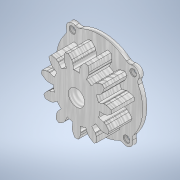
# Autodesk Inventor part: ｍ2歯数10ギアF有d6
Saved by Autodesk Inventor 2020.2 (Build 242310000, 310)
## iProperties
Created: 2020-02-29
Part Number: ｍ2歯数10ギアF有d6
Material: アルミニウム 7075
Document SubType Name: Modeling
Designer: aoyam
Density: 2.81 g/cm^3
Appearance: サテン - ブラシ仕上げ 重厚
Author: aoyam
Autodesk Inventor part; units mm, degrees
ref_plane "YZ Plane" through (0, 0, 0) normal (1, 0, 0) x (0, 1, 0)
ref_plane "XZ Plane" through (0, 0, 0) normal (0, 1, 0) x (-1, 0, 0)
ref_plane "XY Plane" through (0, 0, 0) normal (0, 0, 1) x (1, 0, 0)
sketch "スケッチ1" plane through (0, 0, 0) normal (0, 0, 1) x (1, 0, 0)
  arc A0 (3.44, 13.5335) -> (3.3718, 13.2916) centre (4.6302, 13.067) ccw
  arc A1 (3.8401, 14.2933) -> (3.44, 13.5335) centre (6.7686, 12.2662) ccw
  arc A2 (5.1311, 15.6698) -> (3.8401, 14.2933) centre (9.0569, 10.6941) ccw
  arc A3 (0.735, 13.2916) -> (0.6667, 13.5335) centre (-0.5235, 13.067) ccw
  arc A4 (0.6667, 13.5335) -> (0.2666, 14.2933) centre (-2.6619, 12.2662) ccw
  arc A5 (0.2666, 14.2933) -> (-1.0244, 15.6698) centre (-4.9502, 10.6941) ccw
  arc A6 (3.1375, 11.4699) -> (0.9692, 11.4699) centre (2.0534, 3.0394) ccw
  arc A7 (-1.0244, 15.6698) -> (-2.186, 15.3287) centre (2.0534, 3.0394) ccw
  line L0 (3.1375, 11.4699) -> (3.3718, 13.2916)
  line L1 (0.9692, 11.4699) -> (0.735, 13.2916)
  line L2 (-3.4166, 9.5455) -> (-4.5985, 10.9513)
  arc A8 (-4.5985, 10.9513) -> (-4.7867, 11.1179) centre (-5.5358, 10.082) ccw
  arc A9 (-4.7867, 11.1179) -> (-5.5341, 11.5408) centre (-6.9018, 8.2522) ccw
  arc A10 (-5.5341, 11.5408) -> (-7.3643, 12.0008) centre (-7.9769, 5.6925) ccw
  arc A11 (-7.3643, 12.0008) -> (-8.1571, 11.0858) centre (2.0534, 3.0394) ccw
  arc A12 (-2.4536, 12.6172) -> (-2.3803, 12.3768) centre (-1.2002, 12.8683) ccw
  arc A13 (-1.5925, 10.7178) -> (-3.4166, 9.5455) centre (2.0534, 3.0394) ccw
  line L3 (-1.5925, 10.7178) -> (-2.3803, 12.3768)
  arc A14 (-2.5279, 13.4728) -> (-2.4536, 12.6172) centre (1.0317, 13.3507) ccw
  arc A15 (-2.186, 15.3287) -> (-2.5279, 13.4728) centre (3.8067, 13.2653) ccw
  line L4 (-6.0657, 5.5554) -> (-7.8201, 6.099)
  arc A16 (-7.8201, 6.099) -> (-8.0684, 6.1374) centre (-8.1386, 4.861) ccw
  arc A17 (-8.0684, 6.1374) -> (-8.9258, 6.0892) centre (-8.2984, 2.5831) ccw
  arc A18 (-8.9258, 6.0892) -> (-10.7142, 5.4866) centre (-7.819, -0.1514) ccw
  arc A19 (-10.7142, 5.4866) -> (-10.8865, 4.2883) centre (2.0534, 3.0394) ccw
  arc A20 (-6.9164, 8.6601) -> (-6.7247, 8.4975) centre (-5.9977, 9.549) ccw
  arc A21 (-5.165, 7.5277) -> (-6.0657, 5.5554) centre (2.0534, 3.0394) ccw
  line L5 (-5.165, 7.5277) -> (-6.7247, 8.4975)
  arc A22 (-7.4414, 9.3397) -> (-6.9164, 8.6601) centre (-4.3808, 11.1615) ccw
  arc A23 (-8.1571, 11.0858) -> (-7.4414, 9.3397) centre (-2.0002, 12.5899) ccw
  line L6 (-6.1371, 0.7665) -> (-7.9069, 0.2753)
  arc A24 (-7.9069, 0.2753) -> (-8.1366, 0.1734) centre (-7.5055, -0.9384) ccw
  arc A25 (-8.1366, 0.1734) -> (-8.8318, -0.3308) centre (-6.4085, -2.941) ccw
  arc A26 (-8.8318, -0.3308) -> (-10.0105, -1.8045) centre (-4.5267, -4.9823) ccw
  arc A27 (-10.0105, -1.8045) -> (-9.5076, -2.9058) centre (2.0534, 3.0394) ccw
  arc A28 (-8.5313, 2.9184) -> (-8.2821, 2.8853) centre (-8.239, 4.1629) ccw
  arc A29 (-6.4457, 2.9127) -> (-6.1371, 0.7665) centre (2.0534, 3.0394) ccw
  line L7 (-6.4457, 2.9127) -> (-8.2821, 2.8853)
  arc A30 (-9.3403, 3.2063) -> (-8.5313, 2.9184) centre (-7.7506, 6.3935) ccw
  arc A31 (-10.8865, 4.2883) -> (-9.3403, 3.2063) centre (-6.5201, 8.8823) ccw
  line L8 (-3.6081, -3.3008) -> (-4.8314, -4.6708)
  arc A32 (-4.8314, -4.6708) -> (-4.9695, -4.8808) centre (-3.8376, -5.4748) ccw
  arc A33 (-4.9695, -4.8808) -> (-5.2818, -5.6807) centre (-1.8319, -6.5665) ccw
  arc A34 (-5.2818, -5.6807) -> (-5.4766, -7.5578) centre (0.8547, -7.2664) ccw
  arc A35 (-5.4766, -7.5578) -> (-4.4581, -8.2123) centre (2.0534, 3.0394) ccw
  arc A36 (-6.7856, -2.7848) -> (-6.5581, -2.678) centre (-7.2125, -1.5799) ccw
  arc A37 (-5.028, -1.6621) -> (-3.6081, -3.3008) centre (2.0534, 3.0394) ccw
  line L9 (-5.028, -1.6621) -> (-6.5581, -2.678)
  arc A38 (-7.6219, -2.9801) -> (-6.7856, -2.7848) centre (-8.0077, 0.5607) ccw
  arc A39 (-9.5076, -2.9058) -> (-7.6219, -2.9801) centre (-8.3181, 3.3196) ccw
  line L10 (0.7184, -5.3552) -> (0.43, -7.169)
  arc A40 (0.43, -7.169) -> (0.4273, -7.4203) centre (1.7007, -7.3081) ccw
  arc A41 (0.4273, -7.4203) -> (0.5971, -8.2621) centre (3.9781, -7.1421) ccw
  arc A42 (0.5971, -8.2621) -> (1.448, -9.9465) centre (6.6167, -6.2784) ccw
  arc A43 (1.448, -9.9465) -> (2.6587, -9.9465) centre (2.0534, 3.0394) ccw
  arc A44 (-2.2337, -6.639) -> (-2.1, -6.4261) centre (-3.2443, -5.8561) ccw
  arc A45 (-1.362, -4.7443) -> (0.7184, -5.3552) centre (2.0534, 3.0394) ccw
  line L11 (-1.362, -4.7443) -> (-2.1, -6.4261)
  arc A46 (-2.8316, -7.2553) -> (-2.2337, -6.639) centre (-5.0704, -4.4852) ccw
  arc A47 (-4.4581, -8.2123) -> (-2.8316, -7.2553) centre (-6.8231, -2.3321) ccw
  line L12 (5.4688, -4.7443) -> (6.2067, -6.4261)
  arc A48 (6.2067, -6.4261) -> (6.3404, -6.639) centre (7.351, -5.8561) ccw
  arc A49 (6.3404, -6.639) -> (6.9383, -7.2553) centre (9.1771, -4.4852) ccw
  arc A50 (6.9383, -7.2553) -> (8.5648, -8.2123) centre (10.9298, -2.3321) ccw
  arc A51 (8.5648, -8.2123) -> (9.5833, -7.5578) centre (2.0534, 3.0394) ccw
  arc A52 (3.6794, -7.4203) -> (3.6767, -7.169) centre (2.406, -7.3081) ccw
  arc A53 (3.3883, -5.3552) -> (5.4688, -4.7443) centre (2.0534, 3.0394) ccw
  line L13 (3.3883, -5.3552) -> (3.6767, -7.169)
  arc A54 (3.5096, -8.2621) -> (3.6794, -7.4203) centre (0.1286, -7.1421) ccw
  arc A55 (2.6587, -9.9465) -> (3.5096, -8.2621) centre (-2.51, -6.2784) ccw
  line L14 (9.1347, -1.6621) -> (10.6648, -2.678)
  arc A56 (10.6648, -2.678) -> (10.8923, -2.7848) centre (11.3192, -1.5799) ccw
  arc A57 (10.8923, -2.7848) -> (11.7286, -2.9801) centre (12.1144, 0.5607) ccw
  arc A58 (11.7286, -2.9801) -> (13.6143, -2.9058) centre (12.4248, 3.3196) ccw
  arc A59 (13.6143, -2.9058) -> (14.1172, -1.8045) centre (2.0534, 3.0394) ccw
  arc A60 (9.0762, -4.8808) -> (8.9381, -4.6708) centre (7.9443, -5.4748) ccw
  arc A61 (7.7148, -3.3008) -> (9.1347, -1.6621) centre (2.0534, 3.0394) ccw
  line L15 (7.7148, -3.3008) -> (8.9381, -4.6708)
  arc A62 (9.3885, -5.6807) -> (9.0762, -4.8808) centre (5.9387, -6.5665) ccw
  arc A63 (9.5833, -7.5578) -> (9.3885, -5.6807) centre (3.252, -7.2664) ccw
  line L16 (10.5524, 2.9127) -> (12.3888, 2.8853)
  arc A64 (12.3888, 2.8853) -> (12.638, 2.9184) centre (12.3457, 4.1629) ccw
  arc A65 (12.638, 2.9184) -> (13.447, 3.2063) centre (11.8573, 6.3935) ccw
  arc A66 (13.447, 3.2063) -> (14.9932, 4.2883) centre (10.6269, 8.8823) ccw
  arc A67 (14.9932, 4.2883) -> (14.8209, 5.4866) centre (2.0534, 3.0394) ccw
  arc A68 (12.2433, 0.1734) -> (12.0136, 0.2753) centre (11.6122, -0.9384) ccw
  arc A69 (10.2438, 0.7665) -> (10.5524, 2.9127) centre (2.0534, 3.0394) ccw
  line L17 (10.2438, 0.7665) -> (12.0136, 0.2753)
  arc A70 (12.9385, -0.3308) -> (12.2433, 0.1734) centre (10.5152, -2.941) ccw
  arc A71 (14.1172, -1.8045) -> (12.9385, -0.3308) centre (8.6334, -4.9823) ccw
  line L18 (9.2717, 7.5277) -> (10.8314, 8.4975)
  arc A72 (10.8314, 8.4975) -> (11.0231, 8.6601) centre (10.1044, 9.549) ccw
  arc A73 (11.0231, 8.6601) -> (11.5481, 9.3397) centre (8.4876, 11.1615) ccw
  arc A74 (11.5481, 9.3397) -> (12.2639, 11.0858) centre (6.1069, 12.5899) ccw
  arc A75 (12.2639, 11.0858) -> (11.471, 12.0008) centre (2.0534, 3.0394) ccw
  arc A76 (12.1752, 6.1374) -> (11.9268, 6.099) centre (12.2453, 4.861) ccw
  arc A77 (10.1724, 5.5554) -> (9.2717, 7.5277) centre (2.0534, 3.0394) ccw
  line L19 (10.1724, 5.5554) -> (11.9268, 6.099)
  arc A78 (13.0325, 6.0892) -> (12.1752, 6.1374) centre (12.4051, 2.5831) ccw
  arc A79 (14.8209, 5.4866) -> (13.0325, 6.0892) centre (11.9257, -0.1514) ccw
  line L20 (5.6992, 10.7178) -> (6.487, 12.3768)
  arc A80 (6.487, 12.3768) -> (6.5604, 12.6172) centre (5.3069, 12.8683) ccw
  arc A81 (6.5604, 12.6172) -> (6.6346, 13.4728) centre (3.075, 13.3507) ccw
  arc A82 (6.6346, 13.4728) -> (6.2927, 15.3287) centre (0.3, 13.2653) ccw
  arc A83 (6.2927, 15.3287) -> (5.1311, 15.6698) centre (2.0534, 3.0394) ccw
  arc A84 (8.8934, 11.1179) -> (8.7052, 10.9513) centre (9.6425, 10.082) ccw
  arc A85 (7.5233, 9.5455) -> (5.6992, 10.7178) centre (2.0534, 3.0394) ccw
  line L21 (7.5233, 9.5455) -> (8.7052, 10.9513)
  arc A86 (9.6408, 11.5408) -> (8.8934, 11.1179) centre (11.0085, 8.2522) ccw
  arc A87 (11.471, 12.0008) -> (9.6408, 11.5408) centre (12.0836, 5.6925) ccw
  circle A88 centre (2.0534, 3.0394) radius 3
  circle A89 centre (2.0534, 3.0394) radius 13 construction
  circle A90 centre (-7.9673, 15.5128) radius 1.25
  arc A91 (-6.8532, 17.4676) -> (-10.1163, 14.8461) centre (-7.9673, 15.5128) ccw
  arc A92 (-10.4621, 13.0075) -> (-10.1163, 14.8461) centre (-12.0265, 14.2535) ccw
  arc A93 (-6.8532, 17.4676) -> (-4.9833, 17.409) centre (-5.8629, 19.2052) ccw
  arc A94 (-12.3749, -5.8672) -> (-12.3163, -3.9973) centre (-14.1125, -4.8769) ccw
  circle A95 centre (-10.4201, -6.9813) radius 1.25
  arc A96 (-7.9148, -9.4761) -> (-9.7534, -9.1303) centre (-9.1608, -11.0405) ccw
  arc A97 (-12.3749, -5.8672) -> (-9.7534, -9.1303) centre (-10.4201, -6.9813) ccw
  arc A98 (10.9599, -11.3888) -> (9.09, -11.3302) centre (9.9696, -13.1264) ccw
  circle A99 centre (12.074, -9.434) radius 1.25
  arc A100 (14.5688, -6.9288) -> (14.223, -8.7674) centre (16.1332, -8.1748) ccw
  arc A101 (10.9599, -11.3888) -> (14.223, -8.7674) centre (12.074, -9.434) ccw
  arc A102 (16.4816, 11.9459) -> (16.423, 10.076) centre (18.2192, 10.9556) ccw
  circle A103 centre (14.5268, 13.06) radius 1.25
  arc A104 (12.0215, 15.5548) -> (13.8601, 15.209) centre (13.2675, 17.1192) ccw
  arc A105 (16.4816, 11.9459) -> (13.8601, 15.209) centre (14.5268, 13.06) ccw
  arc A106 (-10.4621, 13.0075) -> (-12.3163, -3.9973) centre (2.0534, 3.0394) ccw
  arc A107 (-7.9148, -9.4761) -> (9.09, -11.3302) centre (2.0534, 3.0394) ccw
  arc A108 (14.5688, -6.9288) -> (16.423, 10.076) centre (2.0534, 3.0394) ccw
  arc A109 (12.0215, 15.5548) -> (-4.9833, 17.409) centre (2.0534, 3.0394) ccw
  point P0 (0, 0)
  point P1 (-5.165, 7.5277)
  point P2 (-6.0657, 5.5554)
  point P3 (-8.0684, 6.1374)
  point P4 (-8.9258, 6.0892)
  point P5 (-10.7142, 5.4866)
  point P6 (-10.8865, 4.2883)
  point P7 (-9.3403, 3.2063)
  point P8 (-8.5313, 2.9184)
  point P9 (-8.2821, 2.8853)
  point P10 (-6.4457, 2.9127)
  point P11 (-6.1371, 0.7665)
  point P12 (-8.1366, 0.1734)
  point P13 (-8.8318, -0.3308)
  point P14 (-10.0105, -1.8045)
  point P15 (-9.5076, -2.9058)
  point P16 (-7.6219, -2.9801)
  point P17 (-6.7856, -2.7848)
  point P18 (-6.5581, -2.678)
  point P19 (-3.6081, -3.3008)
  point P20 (-4.8314, -4.6708)
  point P21 (-4.9695, -4.8808)
  point P22 (-5.2818, -5.6807)
  point P23 (-5.4766, -7.5578)
  point P24 (-4.4581, -8.2123)
  point P25 (-2.8316, -7.2553)
  point P26 (-2.2337, -6.639)
  point P27 (0.7184, -5.3552)
  point P28 (0.43, -7.169)
  point P29 (0.4273, -7.4203)
  point P30 (0.5971, -8.2621)
  point P31 (1.448, -9.9465)
  point P32 (2.6587, -9.9465)
  point P33 (3.5096, -8.2621)
  point P34 (3.6794, -7.4203)
  point P35 (3.6767, -7.169)
  point P36 (3.3883, -5.3552)
  point P37 (6.2067, -6.4261)
  point P38 (6.3404, -6.639)
  point P39 (6.9383, -7.2553)
  point P40 (8.5648, -8.2123)
  point P41 (9.5833, -7.5578)
  point P42 (9.3885, -5.6807)
  point P43 (9.0762, -4.8808)
  point P44 (9.1347, -1.6621)
  point P45 (10.6648, -2.678)
  point P46 (10.8923, -2.7848)
  point P47 (11.7286, -2.9801)
  point P48 (13.6143, -2.9058)
  point P49 (14.1172, -1.8045)
  point P50 (12.9385, -0.3308)
  point P51 (12.2433, 0.1734)
  point P52 (12.0136, 0.2753)
  point P53 (10.2438, 0.7665)
  point P54 (10.5524, 2.9127)
  point P55 (12.638, 2.9184)
  point P56 (13.447, 3.2063)
  point P57 (14.9932, 4.2883)
  point P58 (14.8209, 5.4866)
  point P59 (13.0325, 6.0892)
  point P60 (12.1752, 6.1374)
  point P61 (11.9268, 6.099)
  point P62 (11.0231, 8.6601)
  point P63 (11.5481, 9.3397)
  point P64 (12.2639, 11.0858)
  point P65 (11.471, 12.0008)
  point P66 (9.6408, 11.5408)
  point P67 (8.8934, 11.1179)
  point P68 (6.5604, 12.6172)
  point P69 (6.6346, 13.4728)
  point P70 (6.2927, 15.3287)
  point P71 (5.1311, 15.6698)
  point P72 (3.8401, 14.2933)
  point P73 (3.44, 13.5335)
  point P74 (3.3718, 13.2916)
  point P75 (3.1375, 11.4699)
  point P76 (0.9692, 11.4699)
  point P77 (0.735, 13.2916)
  point P78 (0.6667, 13.5335)
  point P79 (0.2666, 14.2933)
  point P80 (-1.0244, 15.6698)
  point P81 (-2.186, 15.3287)
  point P82 (-2.5279, 13.4728)
  point P83 (-2.4536, 12.6172)
  point P84 (-2.3803, 12.3768)
  point P85 (-4.5985, 10.9513)
  point P86 (-4.7867, 11.1179)
  point P87 (-5.5341, 11.5408)
  point P88 (-7.3643, 12.0008)
  point P89 (-8.1571, 11.0858)
  point P90 (-6.9164, 8.6601)
  point P91 (-6.7247, 8.4975)
  dimension "d2" = 360
  dimension "d4" = 6
  dimension "d6" = 2.5
  dimension "d7" = 1
  dimension "d8" = 2
  dimension "d11" = 360
  dimension "d13" = 16
  constraints: 208 point on circle, 110 centre point, 44 end point, 3 coincident, 2 tangent, 1 equal radius, 462 other
  measures "d4" diameter of A88
  measures "d6" diameter of A90
  measures "d7" radial gap between concentric circles of A90 A91
  measures "d8" radius of A92
  measures "d13" distance of A89.centre A90.centre
extrude "押し出し1" add sketch "スケッチ1" along normal blind 8.5 contours A1 A2 A83 A82 A81 A80 L20 A85 L21 A84 A86 A87 A75 A74 A73 A72 L18 A77 L19 A76 A78 A79 A67 A66 A65 A64 L16 A69 L17 A68 A70 A71 A59 A58 A57 A56 L14 A61 L15 A60 A62 A63 A51 A50 A49 A48 L12 A53 L13 A52 A54 A55 A43 A42 A41 A40 L10 A45 L11 A44 A46 A47 A35 A34 A33 A32 L8 A37 L9 A36 A38 A39 A27 A26 A25 A24 L6 A29 L7 A28 A30 A31 A19 A18 A17 A16 L4 A21 L5 A20 A22 A23 A11 A10 A9 A8 L2 A13 L3 A12 A14 A15 A7 A5 A4 A3 L1 A6 L0 A0
extrude "押し出し2" add sketch "スケッチ1" against normal blind 1.5 contours A1 A2 A83 A82 A81 A80 L20 A85 L21 A84 A86 A87 A75 A74 A73 A72 L18 A77 L19 A76 A78 A79 A67 A66 A65 A64 L16 A69 L17 A68 A70 A71 A59 A58 A57 A56 L14 A61 L15 A60 A62 A63 A51 A50 A49 A48 L12 A53 L13 A52 A54 A55 A43 A42 A41 A40 L10 A45 L11 A44 A46 A47 A35 A34 A33 A32 L8 A37 L9 A36 A38 A39 A27 A26 A25 A24 L6 A29 L7 A28 A30 A31 A19 A18 A17 A16 L4 A21 L5 A20 A22 A23 A11 A10 A9 A8 L2 A13 L3 A12 A14 A15 A7 A5 A4 A3 L1 A6 L0 A0 | A93 A109 A104 A105 A102 A108 A100 A101 A98 A107 A96 A97 A94 A106 A92 A91
thread "ねじ1" size "M3x0.5" class "6H" standard "ANSI Metric M Profile" full length
thread "ねじ2" size "M3x0.5" class "6H" standard "ANSI Metric M Profile" full length
thread "ねじ3" size "M3x0.5" class "6H" standard "ANSI Metric M Profile" full length
thread "ねじ4" size "M3x0.5" class "6H" standard "ANSI Metric M Profile" full length
